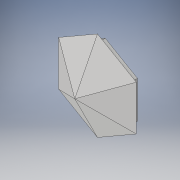
# Autodesk Inventor part: Phage_Hat
Saved by Autodesk Inventor 2019 (Build 230136000, 136)
## iProperties
Created: 2018-09-25
Part Number: Phage_Hat
Material: Generic
Document SubType Name: Modeling
Designer: johan
Density: 1 g/cm^3
Appearance: Default
Author: johan
Autodesk Inventor part; units mm, degrees
ref_plane "YZ Plane" through (0, 0, 0) normal (1, 0, 0) x (0, 1, 0)
ref_plane "XZ Plane" through (0, 0, 0) normal (0, 1, 0) x (-1, 0, 0)
sketch "Sketch1" plane through (0, 0, 0) normal (0, 0, 1) x (1, 0, 0)
  line L0 (-100, 57.735) -> (0, 115.4701)
  line L1 (0, 115.4701) -> (100, 57.735)
  line L2 (100, 57.735) -> (100, -57.735)
  line L3 (100, -57.735) -> (0, -115.4701)
  line L4 (0, -115.4701) -> (-100, -57.735)
  line L5 (-100, -57.735) -> (-100, 57.735)
  line L6 (-95, 54.8483) -> (0, 109.6966)
  line L7 (0, 109.6966) -> (95, 54.8483)
  line L8 (95, 54.8483) -> (95, -54.8483)
  line L9 (95, -54.8483) -> (0, -109.6966)
  line L10 (0, -109.6966) -> (-95, -54.8483)
  line L11 (-95, -54.8483) -> (-95, 54.8483)
  line L12 (-100, -57.735) -> (0, 0)
  line L13 (0, 0) -> (0, -115.4701)
  line L14 (100, -57.735) -> (0, 0)
  line L15 (100, 57.735) -> (0, 0)
  line L16 (0, 115.4701) -> (0, 0)
  line L17 (-100, 57.735) -> (0, 0)
  line L18 (0, -109.6966) -> (0, 0)
  line L19 (95, -54.8483) -> (0, 0)
  line L20 (95, 54.8483) -> (0, 0)
  line L21 (0, 109.6966) -> (0, 0)
  line L22 (-95, 54.8483) -> (0, 0)
  line L23 (-95, -54.8483) -> (0, 0)
  dimension "d0" = 200
  dimension "d1" = 190
  constraints: 48 end point, 6 collinear, 2 coincident, 2 vertical, 26 other
  measures "d0" distance between parallel lines of L5 L2
  measures "d1" distance between parallel lines of L8 L11
ref_plane "Work Plane1" through (0, 0, 58.5) normal (0, 0, 1) x (1, 0, 0)
sketch "Sketch2" plane through (0, 0, 58.5) normal (0, 0, 1) x (1, 0, 0)
  point P0 (0, 0)
  point P1 (0, 0)
  constraints: 1 coincident
extrude "Extrusion1" add sketch "Sketch1" along normal up to surface (58.5 mm away)
loft "Loft1" cut keep common part section 1 edges at (-50, -86.6025, 0) (-100, 0, 0) (-50, 86.6025, 0) (50, 86.6025, 0) (100, 0, 0) (50, -86.6025, 0) section 2 point at (0, 0, 58.5)
shell "Shell1" thickness 10 removed faces 1 at (0, 0, 0)
sketch "Sketch4" plane through (0, 0, 0) normal (0, 0, -1) x (-1, 0, 0)
  line L0 (0, -92.6022) -> (-80.1958, -46.3011) projected
  line L1 (0, -92.6022) -> (-80.1958, -46.3011)
  line L2 (-80.1958, -46.3011) -> (-80.1958, 46.3011)
  line L3 (-80.1958, 46.3011) -> (0, 92.6022)
  line L4 (0, 92.6022) -> (80.1958, 46.3011)
  line L5 (80.1958, 46.3011) -> (80.1958, -46.3011)
  line L6 (80.1958, -46.3011) -> (0, -92.6022)
  line L7 (0, -95.8401) -> (-83, -47.9201)
  line L8 (-83, -47.9201) -> (-83, 47.9201)
  line L9 (-83, 47.9201) -> (0, 95.8401)
  line L10 (0, 95.8401) -> (83, 47.9201)
  line L11 (83, 47.9201) -> (83, -47.9201)
  line L12 (83, -47.9201) -> (0, -95.8401)
  line L13 (83, -47.9201) -> (80.1958, -46.3011)
  line L14 (0, -95.8401) -> (0, -92.6022)
  line L15 (-83, -47.9201) -> (-80.1958, -46.3011)
  line L16 (-83, 47.9201) -> (-80.1958, 46.3011)
  line L17 (0, 95.8401) -> (0, 92.6022)
  line L18 (80.1958, 46.3011) -> (83, 47.9201)
  point P0 (0, 0)
  point P1 (0, 0)
  point P2 (0, 0)
  dimension "d18" = 166
  constraints: 36 end point, 2 coincident, 1 collinear, 1 vertical, 26 other
  measures "d18" distance between parallel lines of L8 L11
extrude "Extrusion3" add sketch "Sketch4" along normal blind 20 contours L14 L7 L15 L0 | L6 L13 L12 L14 | L15 L8 L16 L2 | L5 L18 L11 L13 | L16 L9 L17 L3 | L4 L17 L10 L18
body "Solid1"
